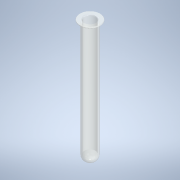
# Autodesk Inventor part: fiolka
Saved by Autodesk Inventor 2021 (Build 250183000, 183)
## iProperties
Created: 2021-05-20
Part Number: fiolka
Material: Szkło
Document SubType Name: Modeling
Designer: Wojciech Wołczek
Density: 2.18 g/cm^3
Appearance: Przezroczyste
Author: Wojciech Wołczek
Autodesk Inventor part; units mm, degrees
ref_plane "YZ Plane" through (0, 0, 0) normal (1, 0, 0) x (0, 1, 0)
ref_plane "XZ Plane" through (0, 0, 0) normal (0, 1, 0) x (-1, 0, 0)
ref_plane "XY Plane" through (0, 0, 0) normal (0, 0, 1) x (1, 0, 0)
sketch "Szkic1" plane through (0, 0, 0) normal (0, 0, 1) x (1, 0, 0)
  line L0 (1, -90) -> (-1, -90)
  line L1 (-10, -81) -> (-10, 90)
  line L2 (-10, 90) -> (-10, 90)
  line L3 (10, 90) -> (10, -81)
  line L4 (10, -90) -> (-10, 90) construction
  line L5 (-10, -90) -> (10, 90) construction
  arc A0 (1, -90) -> (10, -81) centre (1, -81) ccw
  arc A1 (-10, -81) -> (-1, -90) centre (-1, -81) ccw
  line L6 (-10, 90) -> (-14, 90)
  line L7 (-15, 89) -> (-15, 89)
  line L8 (-14, 88) -> (-10, 88)
  line L9 (-10, 88) -> (-10, 90)
  line L10 (10, 90) -> (14, 90)
  line L11 (15, 89) -> (15, 89)
  line L12 (14, 88) -> (10, 88)
  line L13 (10, 88) -> (10, 90)
  arc A2 (14, 88) -> (15, 89) centre (14, 89) ccw
  arc A3 (15, 89) -> (14, 90) centre (14, 89) ccw
  arc A4 (-15, 89) -> (-14, 88) centre (-14, 89) ccw
  arc A5 (-14, 90) -> (-15, 89) centre (-14, 89) ccw
  line L14 (-8, 88) -> (-8, -81)
  arc A6 (-8, -81) -> (-1, -88) centre (-1, -81) ccw
  line L15 (-1, -88) -> (1, -88)
  arc A7 (1, -88) -> (8, -81) centre (1, -81) ccw
  line L16 (8, -81) -> (8, 88)
  arc A8 (-8, 88) -> (-10, 90) centre (-10, 88) ccw
  line L17 (10, 90) -> (10, 90)
  arc A9 (10, 90) -> (8, 88) centre (10, 88) ccw
  line L18 (0, -90) -> (0, 71.327) construction
  line L19 (0, -90) -> (0, -88)
  point P0 (0, 0)
  point P1 (-15, 88)
  point P2 (-15, 90)
  point P3 (15, 88)
  point P4 (-10, 90)
  point P5 (-10, 88)
  dimension "d0" = 20
  dimension "d1" = 180
  dimension "d2" = 9
  dimension "d3" = 9
  dimension "d4" = 5
  dimension "d5" = 2
  dimension "d6" = 5
  dimension "d7" = 1
  dimension "d8" = 1
  dimension "d9" = 1
  dimension "d10" = 1
  dimension "d11" = 2
  dimension "d12" = 2
  dimension "d13" = 2
  constraints: 40 end point, 20 point on circle, 16 tangent, 13 point on line, 10 centre point, 7 parallel, 4 horizontal, 4 midpoint, 4 perpendicular, 1 vertical, 4 other
  measures "d0" distance of L1.end L3.start
  measures "d1" distance of L5.start L1.end
  measures "d2" radius of A0
  measures "d3" radius of A1
  measures "d4" distance of L8.end point (-15, 88)
  measures "d5" distance of point (-15, 88) point (-15, 90)
  measures "d6" distance of point (15, 88) L12.end
  measures "d7" radius of A2
  measures "d8" radius of A3
  measures "d9" radius of A4
  measures "d10" radius of A5
  measures "d11" distance between parallel lines of L1 L14
  measures "d12" radius of A8
  measures "d13" radius of A9
revolve "Obrót1" add sketch "Szkic1" angle 360 about axis through (0, -90, 0) along (0, 1, 0) contours L0 A1 L1 A8 L14 A6 L15 L19 | L8 A4 A5 L6 L1
